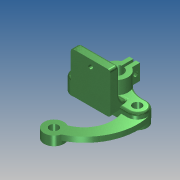
# Autodesk Inventor part: Linearwagen_MauroW_outside_QR-version
Saved by Autodesk Inventor 2015 SP1 (Build 190203100, 203)
## iProperties
Created: 2015-02-25
Part Number: Linearwagen_MauroW_outside_QR-version
Material: Generisch
Document SubType Name: Modeling
Designer: Marc
Density: 1 g/cm^3
Appearance: Gehont - dunkelgrau(2)
Author: Marc
Autodesk Inventor part; units mm, degrees
ref_plane "YZ Plane" through (0, 0, 0) normal (1, 0, 0) x (0, 1, 0)
ref_plane "XZ Plane" through (0, 0, 0) normal (0, 1, 0) x (-1, 0, 0)
ref_plane "XY Plane" through (0, 0, 0) normal (0, 0, 1) x (1, 0, 0)
sketch "Skizze1" plane through (0, 0, 0) normal (0, 0, 1) x (1, 0, 0)
  line L0 (-50.1686, 0) -> (50.7617, 0) projected
  line L1 (0, -73.5762) -> (0, 44.2069) projected
  circle A0 centre (-21, 0) radius 3.3
  circle A1 centre (-21, 0) radius 14.75 construction
  circle A2 centre (21, 0) radius 3.3
  circle A3 centre (21, 0) radius 14.75 construction
  circle A4 centre (0, -42) radius 3.3
  circle A5 centre (0, -42) radius 14.75 construction
  circle A6 centre (0, 5) radius 5.25
  circle A7 centre (0, 5) radius 9
  circle A8 centre (-21, 0) radius 7.5
  circle A9 centre (21, 0) radius 7.5
  arc A10 (-20.3023, 7.4675) -> (-5.7233, 11.9458) centre (-18.4418, 27.3808) ccw
  arc A11 (5.7233, 11.9458) -> (20.3023, 7.4675) centre (18.4418, 27.3808) ccw
  line L2 (-21, -7.5) -> (21, -7.5)
  circle A12 centre (0, -42) radius 7.5
  arc A13 (3.6768, -35.4631) -> (14.5419, -3.8136) centre (-4.4018, -15) ccw
  arc A14 (7.272, -43.8351) -> (28.2692, 1.8462) centre (-10.5, -8) ccw
  point P0 (0, 0)
  point P1 (28.1068, -2.3967)
  point P2 (19.4082, -7.3291)
  point P3 (-19.4082, -7.3291)
  point P4 (13.6211, 1.3423)
  point P5 (2.9103, -48.9123)
  point P6 (28.4986, 0.1465)
  point P7 (-0.3947, -34.5104)
  point P8 (13.9951, -2.6799)
  dimension "d16" = 15
  dimension "d0" = 6.6
  dimension "d3" = 29.5
  dimension "d4" = 21
  dimension "d5" = 6.6
  dimension "d6" = 42
  dimension "d7" = 29.5
  dimension "d12" = 10.5
  dimension "d13" = 18
  dimension "d14" = 5
  dimension "d15" = 15
  dimension "d19" = 20
  dimension "d20" = 20
  dimension "d47" = 15
  dimension "d51" = 22
  dimension "d52" = 40
  dimension "d53" = 27
  dimension "d54" = 34
  constraints: 17 point on circle, 14 centre point, 7 coincident, 3 point on line, 3 tangent, 2 end point, 2 horizontal, 2 symmetric about line, 16 other
  measures "d0" diameter of A0
  measures "d3" diameter of A1
  measures "d4" distance of point (0, 0) A0.centre
  measures "d5" diameter of A4
  measures "d6" distance of point (0, 0) A4.centre
  measures "d7" diameter of A5
  measures "d12" diameter of A6
  measures "d13" diameter of A7
  measures "d14" distance from line of L0 A6.centre
  measures "d15" diameter of A8
  measures "d19" radius of A10
  measures "d20" radius of A11
  measures "d47" diameter of A12
  measures "d51" radius of A13
  measures "d52" radius of A14
  measures "d53" vertical distance of A12.centre A13.centre
  measures "d54" vertical distance of A12.centre A14.centre
extrude "Extrusion1" add sketch "Skizze1" against normal blind 4 contours A0 L0 A8 | L0 A8 A0 | A8 A10 A7 L0 | L0 A7 L1 L2 A8 | A7 L1 A6 L0 | L0 A6 L1 A7 | A7 L0 A9 A13 L2 L1 | L1 A6 L0 A7 | L1 A7 L0 A6 | A7 A11 A9 L0 | A12 L1 A4 | L1 A4 A12 | A13 A9 L2 | L2 A9 L0 A14 A12 A13 | A9 L0 A2 | L0 A2 A9 | A9 A14 L0
extrude "Extrusion2" add sketch "Skizze1" along normal blind 4 contours A0 L0 A8 | L0 A8 A0 | A8 A10 A7 L0 | L0 A7 L1 L2 A8 | A7 L1 A6 L0 | L0 A6 L1 A7 | A7 L0 A9 A13 L2 L1 | L1 A6 L0 A7 | L1 A7 L0 A6 | A7 A11 A9 L0 | A13 A9 L2 | A9 L0 A2 | L0 A2 A9
sketch "Skizze3" plane through (0, 0, 4) normal (0, 0, 1) x (1, 0, 0)
  circle A0 centre (0, 5) radius 5.25 projected
  circle A1 centre (21, 0) radius 3.3 projected
  circle A2 centre (-21, 0) radius 3.3 projected
  line L0 (-21, -7.5) -> (21, -7.5) projected
  arc A3 (21, -7.5) -> (20.3023, 7.4675) centre (21, 0) ccw projected
  arc A4 (5.7233, 11.9458) -> (20.3023, 7.4675) centre (18.4418, 27.3808) ccw projected
  arc A5 (5.7233, 11.9458) -> (-5.7233, 11.9458) centre (0, 5) ccw projected
  arc A6 (-20.3023, 7.4675) -> (-5.7233, 11.9458) centre (-18.4418, 27.3808) ccw projected
  arc A7 (-20.3023, 7.4675) -> (-21, -7.5) centre (-21, 0) ccw projected
  line L1 (0, -64.8762) -> (0, 42.7569) projected
  line L2 (21, -7.5) -> (-21, -7.5) projected
  line L3 (-15, -7.5) -> (15, -7.5)
  line L4 (15, -7.5) -> (15, -13.5)
  line L5 (15, -13.5) -> (-15, -13.5)
  line L6 (-15, -13.5) -> (-15, -7.5)
  point P0 (0, 0)
  point P1 (17.4616, -7.5)
  point P2 (19.488, -7.5)
  dimension "d28" = 30
  dimension "d29" = 6
  constraints: 8 end point, 2 parallel, 1 horizontal, 1 perpendicular, 1 point on line, 1 other
  measures "d28" distance of L4.end L5.end
  measures "d29" distance of L3.end L4.end
extrude "Extrusion3" add sketch "Skizze3" along normal blind 27 and the other way blind 4 contours L1 L5 L6 L0 | L0 L4 L5 L1
sketch "Skizze4" plane through (0, 0, -4) normal (0, 0, -1) x (-1, 0, 0)
  circle A0 centre (-21, 0) radius 3.3 projected
  circle A1 centre (0, 5) radius 5.25 projected
  circle A2 centre (21, 0) radius 3.3 projected
  line L0 (-16.2803, -7.5) -> (21, -7.5) projected
  arc A3 (21, -7.5) -> (20.3023, 7.4675) centre (21, 0) ccw projected
  arc A4 (5.7233, 11.9458) -> (20.3023, 7.4675) centre (18.4418, 27.3808) ccw projected
  arc A5 (5.7233, 11.9458) -> (-5.7233, 11.9458) centre (0, 5) ccw projected
  arc A6 (-20.3023, 7.4675) -> (-5.7233, 11.9458) centre (-18.4418, 27.3808) ccw projected
  arc A7 (-20.3023, 7.4675) -> (-28.2692, 1.8462) centre (-21, 0) ccw projected
  circle A8 centre (-21, 0) radius 7.5
  circle A9 centre (21, 0) radius 7.5
  arc A10 (-7.272, -43.8351) -> (-3.6768, -35.4631) centre (0, -42) ccw projected
  arc A11 (-28.2692, 1.8462) -> (-7.272, -43.8351) centre (10.5, -8) ccw projected
  arc A12 (-16.2803, -7.5) -> (-3.6768, -35.4631) centre (4.4018, -15) ccw projected
  point P0 (0, 0)
  dimension "d34" = 15
  dimension "d35" = 15
  constraints: 2 centre point, 2 coincident
  measures "d34" diameter of A8
  measures "d35" diameter of A9
extrude "Extrusion4" add sketch "Skizze4" along normal blind 3 contours A9 A3 | A7 A8
sketch "Skizze5" plane through (21, 0, -7) normal (0, 0, -1) x (-1, 0, 0)
  circle A0 centre (0, 0) radius 3.3 projected
  circle A1 centre (0, 0) radius 7.5 projected
  circle A2 centre (42, 0) radius 3.3 projected
  circle A3 centre (42, 0) radius 7.5 projected
  circle A4 centre (0, 0) radius 4.5
  circle A5 centre (42, 0) radius 3.3 projected
  circle A6 centre (42, 0) radius 4.5
  point P0 (21, 0)
  dimension "d38" = 9
  dimension "d39" = 9
  constraints: 2 centre point, 2 coincident
  measures "d38" diameter of A4
  measures "d39" diameter of A6
extrude "Extrusion5" add sketch "Skizze5" along normal blind 1 contours A4 | A6
sketch "Skizze6" plane through (-15, -13.5, 31) normal (0, -1, 0) x (1, 0, 0)
  line L0 (30, -31) -> (30, 0) projected
  line L1 (0, 0) -> (30, 0) projected
  line L2 (0, -31) -> (0, 0) projected
  line L3 (30, -31) -> (0, -31) projected
  circle A0 centre (15, -5) radius 1.75
  point P0 (15, -31)
  dimension "d42" = 3.5
  dimension "d43" = 5
  dimension "d44" = 15
  constraints: 1 centre point
  measures "d42" diameter of A0
  measures "d43" distance from line of L1 A0.centre
  measures "d44" distance from line of L2 A0.centre
extrude "Extrusion6" cut sketch "Skizze6" against normal blind 6 contours A0
sketch "Skizze8" plane through (0, 0, -4) normal (0, 0, -1) x (-1, 0, 0)
  circle A0 centre (0, -42) radius 3.3 projected
  circle A1 centre (0, 5) radius 5.25 projected
  arc A2 (-28.2692, 1.8462) -> (-20.3023, 7.4675) centre (-21, 0) ccw projected
  arc A3 (-28.2692, 1.8462) -> (-7.272, -43.8351) centre (10.5, -8) ccw projected
  arc A4 (-7.272, -43.8351) -> (-3.6768, -35.4631) centre (0, -42) ccw projected
  arc A5 (-16.2803, -7.5) -> (-3.6768, -35.4631) centre (4.4018, -15) ccw projected
  line L0 (-16.2803, -7.5) -> (21, -7.5) projected
  arc A6 (20.3023, 7.4675) -> (21, -7.5) centre (21, 0) ccw projected
  arc A7 (5.7233, 11.9458) -> (20.3023, 7.4675) centre (18.4418, 27.3808) ccw projected
  arc A8 (5.7233, 11.9458) -> (-5.7233, 11.9458) centre (0, 5) ccw projected
  arc A9 (-20.3023, 7.4675) -> (-5.7233, 11.9458) centre (-18.4418, 27.3808) ccw projected
  circle A10 centre (0, -42) radius 7.5
  point P0 (0, 0)
  dimension "d55" = 15
  constraints: 1 centre point, 1 coincident
  measures "d55" diameter of A10
extrude "Extrusion7" add sketch "Skizze8" along normal blind 3 contours A10 A4
sketch "Skizze9" plane through (0, -42, -7) normal (0, 0, -1) x (-1, 0, 0)
  circle A0 centre (0, 0) radius 3.3 projected
  circle A1 centre (0, 0) radius 7.5 projected
  circle A2 centre (0, 0) radius 4.5
  point P0 (0, 42)
  dimension "d58" = 9
  constraints: 1 centre point, 1 coincident
  measures "d58" diameter of A2
extrude "Extrusion8" add sketch "Skizze9" along normal blind 1 contours A2
sketch "Skizze10" plane through (0, 0, 4) normal (0, 0, 1) x (1, 0, 0)
  circle A0 centre (0, 5) radius 5.25 projected
  circle A1 centre (0, 5) radius 5.25 projected
  circle A2 centre (21, 0) radius 3.3 projected
  circle A3 centre (-21, 0) radius 3.3 projected
  line L0 (-21, -7.5) -> (-15, -7.5) projected
  line L1 (-15, -7.5) -> (15, -7.5) projected
  line L2 (15, -7.5) -> (21, -7.5) projected
  arc A4 (21, -7.5) -> (20.3023, 7.4675) centre (21, 0) ccw projected
  arc A5 (5.7233, 11.9458) -> (20.3023, 7.4675) centre (18.4418, 27.3808) ccw projected
  arc A6 (5.7233, 11.9458) -> (-5.7233, 11.9458) centre (0, 5) ccw projected
  arc A7 (-20.3023, 7.4675) -> (-5.7233, 11.9458) centre (-18.4418, 27.3808) ccw projected
  arc A8 (-20.3023, 7.4675) -> (-21, -7.5) centre (-21, 0) ccw projected
  circle A9 centre (0, 5) radius 9
  point P0 (0, 0)
  dimension "d61" = 18
  constraints: 1 centre point, 1 coincident, 1 vertical alignment
  measures "d61" diameter of A9
extrude "Extrusion9" add sketch "Skizze10" along normal blind 10 contours A6 A9
sketch "Skizze11" plane through (0, 5, 14) normal (0, 0, 1) x (1, 0, 0)
  circle A0 centre (0, 0) radius 5.25 projected
  circle A1 centre (0, 0) radius 9 projected
  line L0 (0, -68.2) -> (0, 27.7) projected
  line L1 (-4, 7) -> (4, 7)
  line L2 (4, 7) -> (4, 14)
  line L3 (4, 14) -> (-4, 14)
  line L4 (-4, 14) -> (-4, 7)
  line L5 (-40.1, -5) -> (41.1, -5) projected
  point P0 (0, -5)
  dimension "d64" = 8
  dimension "d65" = 7
  dimension "d66" = 7
  constraints: 8 end point, 2 parallel, 1 horizontal, 1 perpendicular, 1 other
  measures "d64" distance of L3.end L2.end
  measures "d65" distance of L2.end L1.end
  measures "d66" distance from line of L1 A0.centre
extrude "Extrusion10" add sketch "Skizze11" against normal blind 12 contours L1 L4 A1 L0 | L0 A1 L2 L1 | L0 L3 L2 A1 | A1 L4 L3 L0
sketch "Skizze12" plane through (0, 0, 14) normal (0, 0, 1) x (1, 0, 0)
  arc A0 (-4, 13.0623) -> (4, 13.0623) centre (0, 5) ccw projected
  line L0 (4, 13.0623) -> (4, 19) projected
  line L1 (4, 19) -> (-4, 19) projected
  line L2 (-4, 19) -> (-4, 13.0623) projected
  circle A1 centre (0, 5) radius 5.25 projected
  line L3 (0, -63.2) -> (0, 32.7) projected
  line L4 (-4, 19) -> (4, 19) projected
  line L5 (-1, 9) -> (1, 9)
  line L6 (1, 9) -> (1, 19)
  line L7 (1, 19) -> (-1, 19)
  line L8 (-1, 19) -> (-1, 9)
  point P0 (0, 0)
  dimension "d69" = 2
  dimension "d70" = 10
  constraints: 8 end point, 2 parallel, 1 horizontal, 1 perpendicular, 1 point on line, 1 other
  measures "d69" distance between parallel lines of L6 L8
  measures "d70" distance between parallel lines of L5 L1
extrude "Extrusion11" cut sketch "Skizze12" against normal blind 12 contours L1 L3 A1 L8 | A1 L3 L5 L8 | L3 A1 L6 L5 | L1 L6 A1 L3 picked at (-0.5563, 9.4024) picked at (0.5563, 9.4024)
sketch "Skizze13" plane through (4, 13.0623, 14) normal (1, 0, 0) x (0, 0, -1)
  line L0 (12, 0) -> (0, 0) projected
  line L1 (12, 5.9377) -> (12, 0) projected
  line L2 (0, 5.9377) -> (12, 5.9377) projected
  line L3 (0, 0) -> (0, 5.9377) projected
  circle A0 centre (6, 2.9377) radius 1.75
  line L4 (12, 5.9377) -> (0, 5.9377) projected
  point P0 (14, -13.0623)
  dimension "d73" = 3.5
  dimension "d74" = 3
  dimension "d75" = 6
  constraints: 1 centre point
  measures "d73" diameter of A0
  measures "d74" distance from line of L4 A0.centre
  measures "d75" distance from line of L3 A0.centre
extrude "Extrusion12" cut sketch "Skizze13" against normal blind 8 contours A0
fillet "Rundung2" radius 9 1 edges at (0, -7.5, 4)
fillet "Rundung3" radius 2 5 edges at (15, -7.5, 22) (15, -4.864, 6.636) (0, -7.5, 31) (-15, -7.5, 22) (-15, -4.864, 6.636)
fillet "Rundung4" radius 2 6 edges at (15, -11.5, 31) (14.4142, -8.0858, 30.4142) (-15, -11.5, 31) (-14.4142, -8.0858, 30.4142) (15, -10.5, 0) (-15, -10.5, 0)
fillet "Rundung6" radius 2 6 edges at (28.4919, 0.3492, 4) (12.5692, 8.2624, 4) (-18, -7.5, 4) (18, -7.5, 4) (-28.4919, 0.3492, 4) (-12.5692, 8.2624, 4)
sketch "Skizze22" plane through (-13, -13.5, 0) normal (0, -1, 0) x (1, 0, 0)
  circle A0 centre (13, 26) radius 1.75 projected
  arc A1 (-2, 2) -> (0, 0) centre (0, 2) ccw projected
  line L0 (26, 0) -> (0, 0) projected
  arc A2 (26, 0) -> (28, 2) centre (26, 2) ccw projected
  line L1 (28, 2) -> (28, 29) projected
  arc A3 (28, 29) -> (26, 31) centre (26, 29) ccw projected
  line L2 (0, 31) -> (26, 31) projected
  arc A4 (0, 31) -> (-2, 29) centre (0, 29) ccw projected
  line L3 (-2, 2) -> (-2, 29) projected
  point P0 (13, 0)
extrude "Extrusion21" add sketch "Skizze22" along normal blind 0.8
equation "\"d5\" = d0"
equation "\"d7\" = d3"
equation "\"d20\" = d19"
